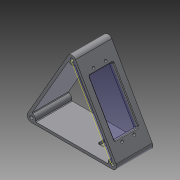
# Autodesk Inventor part: ServoHousing
Saved by Autodesk Inventor 2014 SP1 (Build 180222100, 222)
## iProperties
Created: 2014-11-03
Part Number: ServoHousing
Material: Generic
Document SubType Name: Modeling
Designer: rawrdong
Density: 1 g/cm^3
Appearance: Default
Author: rawrdong
Autodesk Inventor part; units mm, degrees
ref_plane "YZ Plane" through (0, 0, 0) normal (1, 0, 0) x (0, 1, 0)
ref_plane "XZ Plane" through (0, 0, 0) normal (0, 1, 0) x (-1, 0, 0)
ref_plane "XY Plane" through (0, 0, 0) normal (0, 0, 1) x (1, 0, 0)
sketch "Sketch2" plane through (0, 0, 0) normal (0, 1, 0) x (-1, 0, 0)
  circle A0 centre (0, 38.6825) radius 1.425
  circle A1 centre (0, 38.6825) radius 3.5
  circle A2 centre (-33.5, -19.3412) radius 1.425
  circle A3 centre (-33.5, -19.3412) radius 3.5
  circle A4 centre (33.5, -19.3412) radius 1.425
  circle A5 centre (33.5, -19.3412) radius 3.5
  line L0 (-36.5311, -17.5912) -> (-3.0311, 40.4325)
  line L1 (-2.7171, 36.4763) -> (-32.9479, -15.885)
  line L2 (-33.5, -22.8412) -> (33.5, -22.8412)
  line L3 (36.5311, -17.5912) -> (3.0311, 40.4325)
  line L4 (-30.2308, -20.5912) -> (30.2308, -20.5912)
  line L5 (32.9479, -15.885) -> (2.7171, 36.4763)
  line L6 (0, -22.8412) -> (0, -20.5912) construction
  line L7 (19.7811, 11.4206) -> (17.8325, 10.2956) construction
  line L8 (-17.8325, 10.2956) -> (-19.7811, 11.4206) construction
  point P0 (0, 0)
  point P1 (0, 0)
  dimension "d21" = 360
  dimension "d23" = 67
  dimension "d24" = 2.85
  dimension "d25" = 7
  dimension "d30" = 2.25
  constraints: 18 end point, 12 point on circle, 6 centre point, 6 midpoint, 6 tangent, 4 coincident, 3 parallel, 2 equal length, 1 horizontal, 1 vertical alignment, 13 other
  measures "d23" distance of A4.centre A2.centre
  measures "d24" diameter of A2
  measures "d25" diameter of A3
  measures "d30" distance between parallel lines of L0 L1
extrude "Extrusion3" add sketch "Sketch2" along normal blind 30 contours A1 | A1 L3 A5 L5 | A1 L1 A3 L0 | A5 | A3 | A5 L2 A3 L4
sketch "Servo1" plane through (36.5311, 0, -17.5912) normal (0.8660254, 0, 0.5) x (0.5, 0, -0.8660254)
  line L0 (-67, 30) -> (0, 30) projected
  line L1 (-54.5, 24.9) -> (-12.5, 24.9)
  line L2 (-12.5, 24.9) -> (-12.5, 5.1)
  line L3 (-12.5, 5.1) -> (-54.5, 5.1)
  line L4 (-54.5, 5.1) -> (-54.5, 24.9)
  circle A0 centre (-9.87, 20) radius 1.075
  circle A1 centre (-9.87, 10) radius 1.075
  line L5 (-33.5, 30) -> (-33.5, -15.5284)
  line L6 (-12.5, 15) -> (-54.5, 15) construction
  circle A2 centre (-57.13, 20) radius 1.075
  circle A3 centre (-57.13, 10) radius 1.075
  line L7 (0, 0) -> (0, 30) projected
  point P0 (-33.5, 0)
  point P1 (-33.5, 5.1)
  point P2 (0, 15)
  dimension "d43" = 2.15
  dimension "d44" = 19.8
  dimension "d45" = 42
  dimension "d47" = 47.26
  dimension "d96" = 10
  constraints: 12 end point, 5 midpoint, 4 centre point, 3 parallel, 3 symmetric about line, 1 equal radius, 1 horizontal, 1 horizontal alignment, 1 perpendicular, 1 point on line, 2 other
  measures "d43" diameter of A0
  measures "d44" distance of L3.end L1.start
  measures "d45" distance of L2.end L3.end
  measures "d47" diameter of A0.centre L5
  measures "d96" distance of A0.centre A1.centre
extrude "Extrusion4" cut sketch "Servo1" against normal blind 27 contours L1 L5 L3 L4 | L1 L2 L3 L5
extrude "Extrusion5" cut sketch "Servo1" against normal up to next contours A0 | A1 | A2 | A3
fillet "Fillet4" radius 0.8 4 edges at (8.3068, 24.9, 29.0447) (8.3068, 5.1, 29.0447) (29.3068, 5.1, -7.3284) (29.3068, 24.9, -7.3284)
ref_plane "Work Plane1" through (2.7171, 0, 36.4763) normal (-0.8660254, 0, -0.5) x (-0.5, 0, 0.8660254)
sketch "Sketch7" plane through (2.7171, 0, 36.4763) normal (-0.8660254, 0, -0.5) x (-0.5, 0, 0.8660254)
  line L0 (-9.2308, 5.9) -> (-9.2308, 24.1) projected
  line L1 (-10.0308, 24.9) -> (-50.4308, 24.9) projected
  arc A0 (-9.2308, 24.1) -> (-10.0308, 24.9) centre (-10.0308, 24.1) ccw projected
  arc A1 (-10.0308, 5.1) -> (-9.2308, 5.9) centre (-10.0308, 5.9) ccw projected
  line L2 (-50.4308, 5.1) -> (-10.0308, 5.1) projected
  arc A2 (-51.2308, 5.9) -> (-50.4308, 5.1) centre (-50.4308, 5.9) ccw projected
  line L3 (-51.2308, 24.1) -> (-51.2308, 5.9) projected
  arc A3 (-50.4308, 24.9) -> (-51.2308, 24.1) centre (-50.4308, 24.1) ccw projected
  line L4 (-50.4308, 27.4) -> (-10.0308, 27.4)
  arc A4 (-6.7308, 24.1) -> (-10.0308, 27.4) centre (-10.0308, 24.1) ccw
  line L5 (-6.7308, 24.1) -> (-6.7308, 5.9)
  arc A5 (-10.0308, 2.6) -> (-6.7308, 5.9) centre (-10.0308, 5.9) ccw
  line L6 (-10.0308, 2.6) -> (-50.4308, 2.6)
  arc A6 (-53.7308, 5.9) -> (-50.4308, 2.6) centre (-50.4308, 5.9) ccw
  line L7 (-53.7308, 5.9) -> (-53.7308, 24.1)
  arc A7 (-50.4308, 27.4) -> (-53.7308, 24.1) centre (-50.4308, 24.1) ccw
  line L8 (-53.7308, 24.1) -> (-62.6767, 24.1)
  line L9 (-62.6767, 24.1) -> (-62.6767, 5.9)
  line L10 (-53.7308, 5.9) -> (-62.6767, 5.9)
  line L11 (-30.2308, 5.1) -> (-30.2308, 24.9) construction
  line L12 (-6.7308, 24.1) -> (2.2151, 24.1)
  line L13 (2.2151, 24.1) -> (2.2151, 5.9)
  line L14 (-6.7308, 5.9) -> (2.2151, 5.9)
  circle A8 centre (-53.8608, 20) radius 1.075 projected
  circle A9 centre (-53.8608, 10) radius 1.075 projected
  circle A10 centre (-6.6008, 10) radius 1.075 projected
  circle A11 centre (-6.6008, 20) radius 1.075 projected
  dimension "d82" = 2.5
  constraints: 22 end point, 8 point on circle, 4 centre point, 3 perpendicular, 2 horizontal, 2 midpoint, 1 vertical, 8 other
  measures "d82" distance between parallel lines of L4 L1
extrude "Extrusion8" add sketch "Sketch7" along normal blind 2 contours L4 A4 L5 A11 A10 A5 L6 A6 L7 A9 A8 A7 | L7 A8 A9 L10 L9 L8 | L12 L13 L14 L5 A10 A11
fillet "Fillet6" radius 2 4 edges at (28.7165, 24.1, -10.556) (5.2165, 24.1, 30.1472) (5.2165, 5.9, 30.1472) (28.7165, 5.9, -10.556)
chamfer "Chamfer2" distance 2 angle 45 14 edges at (17.8325, 27.4, 10.2956) (6.8119, 26.8386, 29.3839) (5.8364, 24.4403, 31.0735) (3.9978, 24.1, 34.2581) (28.8532, 26.8386, -8.7927) (29.8286, 24.4403, -10.4823) (31.6673, 24.1, -13.6669) (17.8325, 2.6, 10.2956) (28.8532, 3.1614, -8.7927) (29.8286, 5.5597, -10.4823) (31.6673, 5.9, -13.6669) (6.8119, 3.1614, 29.3839) (5.8364, 5.5597, 31.0735) (3.9978, 5.9, 34.2581)
fillet "Fillet7" radius 0.5 8 edges at (2.7171, 1.9501, 36.4763) (-2.7171, 15, 36.4763) (2.7171, 28.05, 36.4763) (-32.9479, 15, -15.885) (-30.2308, 15, -20.5912) (30.2308, 15, -20.5912) (32.9479, 1.95, -15.885) (32.9479, 28.0499, -15.885)
chamfer "Chamfer3" distance 0.5 angle 45 8 edges at (19.7811, 5.1, 11.4206) (9.3982, 5.3343, 29.4042) (9.2811, 15, 29.6072) (9.3982, 24.6657, 29.4042) (19.7811, 24.9, 11.4206) (30.1639, 24.6657, -6.563) (30.2811, 15, -6.7659) (30.1639, 5.3343, -6.563)
sketch "Sketch9" plane through (33.5, 0, -22.8412) normal (0, 0, -1) x (-1, 0, 0)
  line L0 (0, 0) -> (0, 30)
  line L1 (17.5, 20) -> (22.5, 20)
  line L2 (22.5, 20) -> (22.5, 10)
  line L3 (22.5, 10) -> (17.5, 10)
  line L4 (17.5, 10) -> (17.5, 20)
  line L5 (0, 15) -> (22.5, 15) construction
  point P0 (-33.5, 0)
  dimension "d97" = 5
  dimension "d98" = 10
  dimension "d104" = 22.5
  constraints: 12 end point, 2 horizontal, 2 midpoint, 2 parallel, 1 perpendicular
  measures "d97" distance of L1.start L1.end
  measures "d98" distance of L3.end L1.start
  measures "d104" distance of L5.start L5.end
extrude "Extrusion9" cut sketch "Sketch9" against normal up to surface surface through (-2.7171, 0, 36.4763) normal (0.8660254, 0, -0.5)
fillet "Fillet8" radius 1.5 4 edges at (11, 20, -21.7162) (16, 20, -21.7162) (16, 10, -21.7162) (11, 10, -21.7162)
body "Solid2"
body "Solid3"
